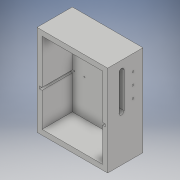
# Autodesk Inventor part: body
Saved by Autodesk Inventor 2019 (Build 230136000, 136)
## iProperties
Created: 2018-06-15
Part Number: body
Material: Generic
Document SubType Name: Modeling
Designer: daniel
Density: 1 g/cm^3
Appearance: Default
Author: daniel
Autodesk Inventor part; units mm, degrees
ref_plane "YZ Plane" through (0, 0, 0) normal (1, 0, 0) x (0, 1, 0)
ref_plane "XZ Plane" through (0, 0, 0) normal (0, 1, 0) x (-1, 0, 0)
ref_plane "XY Plane" through (0, 0, 0) normal (0, 0, 1) x (1, 0, 0)
sketch "Sketch3" plane through (0, 0, 0) normal (0, 0, 1) x (1, 0, 0)
  line L0 (-70, -90) -> (70, -90)
  line L1 (70, -90) -> (70, 90)
  line L2 (70, 90) -> (-70, 90)
  line L3 (-70, 90) -> (-70, -90)
  line L4 (-70, -90) -> (70, 90) construction
  line L5 (70, -90) -> (-70, 90) construction
  point P0 (0, 0)
  dimension "d7" = 140
  dimension "d8" = 180
  constraints: 12 end point, 2 midpoint, 2 parallel, 1 horizontal, 1 perpendicular
  measures "d7" distance of L2.end L1.end
  measures "d8" distance of L1.end L0.end
extrude "Extrusion3" add sketch "Sketch3" along normal blind 70
shell "Shell2" thickness 10 removed faces 1 at (-23.3333, 30, 70)
sketch "Sketch4" plane through (0, 0, 70) normal (0, 0, 1) x (1, 0, 0)
  line L0 (-98, 0) -> (98, 0) projected
  line L1 (0, 126) -> (0, -126) projected
  line L2 (-65, -13) -> (65, -13)
  line L3 (65, -13) -> (65, -8)
  line L4 (65, -8) -> (-65, -8)
  line L5 (-65, -8) -> (-65, -13)
  line L6 (-65, -13) -> (65, -8) construction
  line L7 (65, -13) -> (-65, -8) construction
  line L8 (-60, 80) -> (60, 80) projected
  line L9 (-70, 90) -> (-70, -90) projected
  point P0 (0, 0)
  point P1 (0, -10.5)
  dimension "d12" = 5
  dimension "d13" = 88
  dimension "d19" = 5
  constraints: 12 end point, 2 midpoint, 2 parallel, 1 horizontal, 1 perpendicular, 1 point on line
  measures "d12" distance of L3.end L2.end
  measures "d13" distance between parallel lines of L8 L4
  measures "d19" distance between parallel lines of L9 L5
extrude "Extrusion4" cut sketch "Sketch4" against normal up to surface (60 mm away)
sketch "Sketch6" plane through (-60, -80, 10) normal (0, 0, 1) x (1, 0, 0)
  line L0 (-5, 72) -> (0, 72) projected
  line L1 (0, 72) -> (0, 160) projected
  point P0 (60, 80)
  point P1 (4, 72)
  point P2 (24, 72)
  dimension "d20" = 20
  dimension "d21" = 4
  constraints: 2 point on line
  measures "d20" distance of point (4, 72) point (24, 72)
  measures "d21" distance from line of L1 point (4, 72)
hole "Hole1" at (-56, -8, 10) at (-36, -8, 10) direction (0, 0, -1) diameter 2.4 end through all clearance for "Countersunk Flat Head Screw DIN EN ISO 2009" size "M2" standard "DIN"
sketch "Sketch7" plane through (60, 80, 10) normal (-1, 0, 0) x (0, 0, 1)
  line L0 (60, -88) -> (0, -88) projected
  line L1 (0, -86.8) -> (0, -89.2) projected
  line L2 (0, -86.8) -> (0, -89.2) projected
  line L3 (0, -93) -> (0, -160) projected
  line L4 (0, -160) -> (0, -93) projected
  line L5 (0, -88) -> (0, -93) projected
  line L6 (0, -88) -> (0, 0) projected
  line L7 (0, 0) -> (0, -88) projected
  line L8 (0, -93) -> (0, -88) projected
  line L9 (10, -44) -> (10, -54) construction
  point P0 (-10, -80)
  point P1 (10, -21)
  point P2 (10, -67)
  dimension "d29" = 44
  dimension "d30" = 23
  dimension "d31" = 46
  dimension "d33" = 10
  dimension "d34" = 10
  constraints: 2 end point, 2 point on line, 1 vertical
  measures "d29" distance from line of L0 L9.start
  measures "d30" distance of L9.start point (10, -21)
  measures "d31" distance of point (10, -67) point (10, -21)
  measures "d33" distance from line of L6 L9.start
  measures "d34" distance of L9.start L9.end
hole "Hole2" at (60, 36, 20) at (60, 59, 20) at (60, 13, 20) direction (1, 0, 0) diameter 3.4 end through all clearance for "Countersunk Flat Head Screw DIN EN ISO 2009" size "M3" standard "DIN"
sketch "Sketch8" plane through (70, -90, 0) normal (1, 0, 0) x (0, 0, -1)
  circle A0 centre (-20, 126) radius 1.7 projected
  line L0 (-37.5, 86) -> (-47.5, 86)
  line L1 (-47.5, 86) -> (-47.5, 166)
  line L2 (-47.5, 166) -> (-37.5, 166)
  line L3 (-37.5, 166) -> (-37.5, 86)
  line L4 (-37.5, 86) -> (-47.5, 166) construction
  line L5 (-47.5, 86) -> (-37.5, 166) construction
  line L6 (0, 0) -> (0, 180) projected
  line L7 (-42.5, 126) -> (-20, 126) construction
  point P0 (0, 90)
  dimension "d42" = 37.5
  dimension "d43" = 80
  dimension "d44" = 10
  constraints: 14 end point, 2 horizontal, 2 midpoint, 2 parallel, 1 perpendicular
  measures "d42" distance between parallel lines of L6 L3
  measures "d43" distance of L0.end L1.end
  measures "d44" distance of L1.end L2.end
extrude "Extrusion6" cut sketch "Sketch8" against normal up to surface (10 mm away) contours L0 L1 L2 L3
full round fillet "Fillet1" first side at (66.6667, 49.3333, 37.5) centre faces at (66.6667, -4, 40.8333) second side at (66.6667, 22.6667, 47.5)
full round fillet "Fillet2" first side at (66.6667, 25.9999, 37.5) centre faces at (66.6667, 76, 44.1667) second side at (66.6667, 25.9999, 47.5)
body "Solid1"
body "Solid2"
